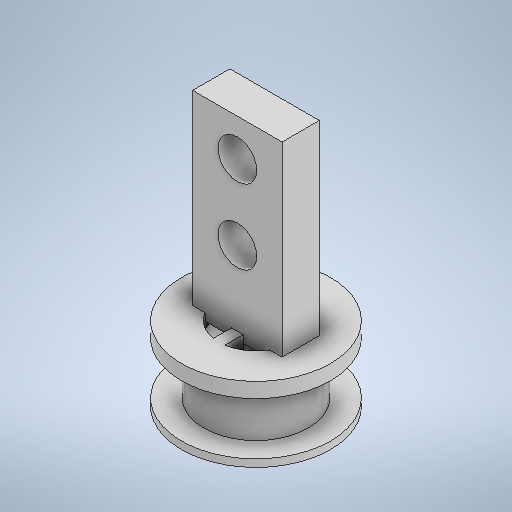
# Autodesk Inventor part: 圓形同心線圈外
Saved by Autodesk Inventor 2025.2 (Build 292293000, 293)
## iProperties
Created: 2025-07-24
Part Number: 圓形同心線圈外
Material: 一般
Document SubType Name: Modeling
Designer: 123
Density: 1 g/cm^3
Appearance: 預設
Author: 123
Autodesk Inventor part; units mm, degrees
ref_plane "YZ Plane" through (0, 0, 0) normal (1, 0, 0) x (0, 1, 0)
ref_plane "XZ Plane" through (0, 0, 0) normal (0, 1, 0) x (-1, 0, 0)
ref_plane "XY Plane" through (0, 0, 0) normal (0, 0, 1) x (1, 0, 0)
sketch "草圖1" plane through (0, 0, 0) normal (0, 1, 0) x (-1, 0, 0)
  line L0 (6, 2.5) -> (-6, 2.5)
  line L1 (-6, 2.5) -> (-6, -2.5)
  line L2 (-6, -2.5) -> (6, -2.5)
  line L3 (6, -2.5) -> (6, 2.5)
  line L4 (6, 2.5) -> (-6, -2.5) construction
  line L5 (-6, 2.5) -> (6, -2.5) construction
  point P0 (0, 0)
  dimension "d0" = 5
  dimension "d1" = 12
  constraints: 12 end point, 2 midpoint, 2 parallel, 1 horizontal, 1 perpendicular
  measures "d0" distance of L2.end L0.start
  measures "d1" distance of L1.end L2.end
extrude "擠出1" add sketch "草圖1" along normal blind 25
sketch "草圖2" plane through (-6, 0, 2.5) normal (0, 0, 1) x (1, 0, 0)
  circle A0 centre (6, 20) radius 2.6
  circle A1 centre (6, 10) radius 2.6
  line L0 (0, 0) -> (12, 0) projected
  line L1 (0, 25) -> (12, 25) projected
  line L2 (6, 25) -> (6, 0)
  line L3 (12, 0) -> (0, 0) projected
  point P0 (6, 0)
  dimension "d4" = 5.2
  dimension "d5" = 5.2
  dimension "d6" = 10
  dimension "d7" = 10
  dimension "d8" = 5
  constraints: 2 centre point, 2 end point, 2 midpoint, 1 perpendicular
  measures "d4" diameter of A0
  measures "d5" diameter of A1
  measures "d6" distance of L2.end A1.centre
  measures "d7" distance of A1.centre A0.centre
  measures "d8" distance from line of L1 A0.centre
extrude "擠出2" cut sketch "草圖2" against normal blind 10
sketch "草圖3" plane through (0, 0, 0) normal (0, -1, 0) x (1, 0, 0)
  circle A0 centre (0, 0) radius 5
  circle A1 centre (0, 0) radius 10
  dimension "d11" = 10
  dimension "d12" = 20
  constraints: 2 centre point, 2 coincident
  measures "d11" diameter of A0
  measures "d12" diameter of A1
extrude "擠出3" add sketch "草圖3" along normal blind 2
sketch "草圖4" plane through (0, -2, 0) normal (0, -1, 0) x (1, 0, 0)
  circle A0 centre (0, 0) radius 6
  circle A1 centre (0, 0) radius 7
  dimension "d15" = 12
  dimension "d16" = 14
  constraints: 2 centre point, 2 coincident
  measures "d15" diameter of A0
  measures "d16" diameter of A1
extrude "擠出4" add sketch "草圖4" along normal blind 7
sketch "草圖5" plane through (0, 0, 0) normal (0, -1, 0) x (1, 0, 0)
  line L0 (-1.5, 1) -> (1.5, 1)
  line L1 (1.5, 1) -> (1.5, -1)
  line L2 (1.5, -1) -> (-1.5, -1)
  line L3 (-1.5, -1) -> (-1.5, 1)
  line L4 (-1.5, 1) -> (1.5, -1) construction
  line L5 (1.5, 1) -> (-1.5, -1) construction
  point P0 (0, 0)
  dimension "d19" = 3
  dimension "d20" = 2
  constraints: 12 end point, 2 midpoint, 2 parallel, 1 horizontal, 1 perpendicular
  measures "d19" distance of L0.start L0.end
  measures "d20" distance of L0.end L1.end
extrude "擠出5" add sketch "草圖5" along normal blind 7
sketch "草圖6" plane through (0, 0, 0) normal (0, 1, 0) x (1, 0, 0)
  line L0 (-4.3301, -2.5) -> (4.3301, -2.5) projected
  line L1 (-0.7875, -7.5) -> (0.7875, -7.5)
  line L2 (0.7875, -7.5) -> (0.7875, -2.5)
  line L3 (0.7875, -2.5) -> (-0.7875, -2.5)
  line L4 (-0.7875, -2.5) -> (-0.7875, -7.5)
  arc A0 (-4.3301, -2.5) -> (4.3301, -2.5) centre (0, 0) ccw projected
  line L5 (-0.7875, -7.5) -> (0.7875, -2.5) construction
  line L6 (0.7875, -7.5) -> (-0.7875, -2.5) construction
  line L7 (-0.7875, 7.5) -> (0.7875, 7.5)
  line L8 (0.7875, 7.5) -> (0.7875, 2.5)
  line L9 (0.7875, 2.5) -> (-0.7875, 2.5)
  line L10 (-0.7875, 2.5) -> (-0.7875, 7.5)
  arc A1 (4.3301, 2.5) -> (-4.3301, 2.5) centre (0, 0) ccw projected
  line L11 (-0.7875, 7.5) -> (0.7875, 2.5) construction
  line L12 (0.7875, 7.5) -> (-0.7875, 2.5) construction
  point P0 (0, -5)
  point P1 (0, 5)
  constraints: 24 end point, 4 midpoint, 4 parallel, 2 horizontal, 2 perpendicular, 2 point on circle, 2 point on line
extrude "擠出6" add sketch "草圖6" against normal blind 2 contours L0 L2 A0 L4 | A0 L2 L1 L4 | L7 L8 A1 L10 | A1 L8 L9 L10
sketch "草圖7" plane through (0, -9, 0) normal (0, -1, 0) x (1, 0, 0)
  circle A0 centre (0, 0) radius 6
  circle A1 centre (0, 0) radius 10
  constraints: 2 centre point, 2 coincident
extrude "擠出7" add sketch "草圖7" along normal blind 1
sketch "草圖8" plane through (0, 0, 0) normal (0, -1, 0) x (1, 0, 0)
  line L0 (4.3301, 2.5) -> (6, 2.5) projected
  line L1 (-6, -2.5) -> (6, -2.5)
  line L2 (6, -2.5) -> (6, 2.5)
  line L3 (6, 2.5) -> (-6, 2.5)
  line L4 (-6, 2.5) -> (-6, -2.5)
  line L5 (-6, -2.5) -> (6, 2.5) construction
  line L6 (6, -2.5) -> (-6, 2.5) construction
  point P0 (0, 0)
  constraints: 12 end point, 2 midpoint, 2 parallel, 1 horizontal, 1 perpendicular
extrude "擠出8" add sketch "草圖8" along normal blind 1
equation "\"d9\" = d7"
